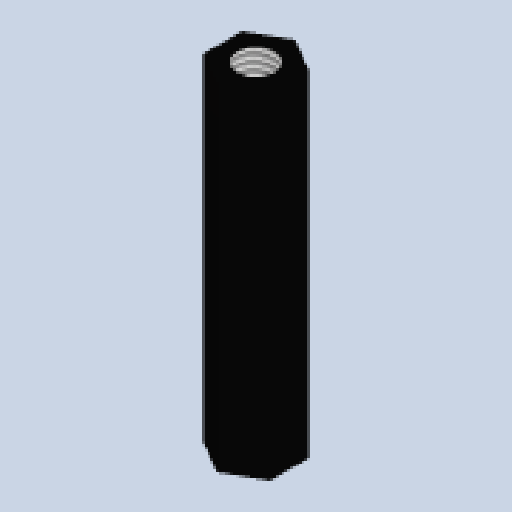
# Autodesk Inventor part: Standoff
Saved by Autodesk Inventor 2024 (Build 280153000, 153)
## iProperties
Created: 2023-11-20
Part Number: Standoff
Material: Aluminum 6061
Document SubType Name: Modeling
Designer: Greg
Density: 2.7 g/cm^3
Appearance: Aluminum - Flat
Author: Greg
Autodesk Inventor part; units mm, degrees
ref_plane "YZ Plane" through (0, 0, 0) normal (1, 0, 0) x (0, 1, 0)
ref_plane "XZ Plane" through (0, 0, 0) normal (0, 1, 0) x (-1, 0, 0)
ref_plane "XY Plane" through (0, 0, 0) normal (0, 0, 1) x (1, 0, 0)
sketch "Sketch1" plane through (0, 0, 0) normal (0, 1, 0) x (-1, 0, 0)
  line L0 (-2.25, -1.299) -> (-2.25, 1.299)
  line L1 (-2.25, 1.299) -> (0, 2.5981)
  line L2 (0, 2.5981) -> (2.25, 1.299)
  line L3 (2.25, 1.299) -> (2.25, -1.299)
  line L4 (2.25, -1.299) -> (0, -2.5981)
  line L5 (0, -2.5981) -> (-2.25, -1.299)
  point P0 (0, 0)
  point P1 (0, 0)
  dimension "d0" = 4.5
  constraints: 12 end point, 1 coincident, 1 vertical, 13 other
  measures "d0" distance between parallel lines of L0 L3
extrude "Extrusion1" add sketch "Sketch1" along normal blind 26.25
sketch "Sketch2" plane through (0, 26.25, 0) normal (0, 1, 0) x (1, 0, 0)
  point P0 (0, 0)
  point P1 (0, 0)
  constraints: 1 coincident
hole "Hole1" at (0, 26.25, 0) direction (0, -1, 0) diameter 2.459 end through all thread size "M3x0.5" class "6H" standard "ISO Metric profile"
body "Solid1"
